Autodesk Fusion 360 part; units mm, degrees
note: some values were not read from the file. Set by a fixed rule: which sketch regions a step uses.
(part 14 of 15)
  line L11464 (261.515, -47.6876) -> (261.464, -47.4097)
  line L11465 (-56.9781, -48.1712) -> (-56.8353, -48.2894)
  line L11466 (-56.8353, -48.2894) -> (-56.7181, -48.4331)
  line L11467 (-57.5292, -49.9086) -> (-57.7133, -49.8866)
  line L11468 (-57.6874, -48.0256) -> (-57.5027, -48.0088)
  line L11469 (-57.7133, -49.8866) -> (-57.8897, -49.8293)
  line L11470 (264.04, -45.2787) -> (264.303, -45.3806)
  line L11471 (263.765, -45.2149) -> (264.04, -45.2787)
  line L11472 (-58.4437, -49.1303) -> (-58.4593, -48.9455)
  line L11473 (-56.631, -48.5968) -> (-56.5774, -48.7743)
  line L11474 (-57.1658, -49.8445) -> (-57.3444, -49.8943)
  line L11475 (-56.5593, -48.9588) -> (-56.5597, -48.9853)
  line L11476 (-58.4593, -48.9455) -> (-58.4386, -48.7613)
  line L11477 (-58.0295, -48.1639) -> (-57.8652, -48.078)
  line L11478 (94.3983, -48.4103) -> (94.5428, -48.2941)
  line L11479 (95.9894, -49.2995) -> (95.9308, -49.4755)
  line L11480 (264.775, -45.69) -> (264.973, -45.8914)
  line L11481 (-57.8897, -49.8293) -> (-58.0515, -49.7389)
  line L11482 (-57.3183, -48.0282) -> (-57.1412, -48.083)
  line L11483 (94.2791, -48.5523) -> (94.3983, -48.4103)
  line L11484 (72.3389, -48.542) -> (72.1284, -48.7305)
  line L11485 (261.453, -47.1274) -> (261.482, -46.8464)
  line L11486 (261.973, -45.8442) -> (262.177, -45.6492)
  line L11487 (263.201, -45.206) -> (263.483, -45.1905)
  line L11488 (264.678, -48.7706) -> (264.443, -48.9275)
  line L11489 (72.1284, -48.7305) -> (71.8935, -48.8875)
  line L11490 (265.432, -46.9085) -> (265.452, -47.1903)
  line L11491 (71.3695, -49.0949) -> (71.0908, -49.1413)
  line L11492 (69.9946, -48.9322) -> (69.7526, -48.7865)
  line L11493 (69.7526, -48.7865) -> (69.5335, -48.6081)
  line L11494 (72.9026, -47.1502) -> (72.8987, -47.2758)
  line L11495 (69.1811, -48.1683) -> (69.0548, -47.9156)
  line L11496 (69.1066, -46.2703) -> (69.2484, -46.026)
  line L11497 (262.924, -45.2612) -> (263.201, -45.206)
  line L11498 (265.141, -46.1186) -> (265.275, -46.3672)
  line L11499 (72.8232, -46.5922) -> (72.8827, -46.8684)
  line L11500 (262.177, -45.6492) -> (262.407, -45.485)
  line L11501 (265.275, -46.3672) -> (265.372, -46.6323)
  line L11502 (262.407, -45.485) -> (262.658, -45.3548)
  line L11503 (262.302, -48.8266) -> (262.083, -48.6482)
  line L11504 (70.1083, -45.3147) -> (70.3749, -45.2211)
  line L11505 (70.5278, -49.1148) -> (70.2548, -49.0424)
  line L11506 (70.6519, -45.166) -> (70.934, -45.1505)
  line L11507 (265.334, -47.8677) -> (265.219, -48.1261)
  line L11508 (71.7542, -45.3406) -> (72.0007, -45.4786)
  line L11509 (263.483, -45.1905) -> (263.765, -45.2149)
  line L11510 (72.8827, -46.8684) -> (72.9026, -47.1502)
  line L11511 (72.2252, -45.65) -> (72.4234, -45.8513)
  line L11512 (262.544, -48.9723) -> (262.302, -48.8266)
  line L11513 (70.8084, -49.148) -> (70.5278, -49.1148)
  line L11514 (68.9324, -46.8063) -> (69.0005, -46.5322)
  line L11515 (72.7254, -46.3272) -> (72.8232, -46.5922)
  line L11516 (258.64, -47.1418) -> (258.817, -47.1966)
  line L11517 (69.4233, -45.8042) -> (69.6278, -45.6092)
  line L11518 (68.9654, -47.6476) -> (68.9147, -47.3697)
  line L11519 (70.934, -45.1505) -> (71.2155, -45.1748)
  line L11520 (264.188, -49.0498) -> (263.919, -49.135)
  line L11521 (265.372, -46.6323) -> (265.432, -46.9085)
  line L11522 (72.4234, -45.8513) -> (72.5913, -46.0785)
  line L11523 (265.07, -48.3658) -> (264.888, -48.5821)
  line L11524 (71.8935, -48.8875) -> (71.6389, -49.0098)
  line L11525 (71.6389, -49.0098) -> (71.3695, -49.0949)
  line L11526 (261.656, -46.3104) -> (261.798, -46.0661)
  line L11527 (71.2155, -45.1748) -> (71.4907, -45.2386)
  line L11528 (72.7844, -47.8277) -> (72.6701, -48.0861)
  line L11529 (71.0908, -49.1413) -> (70.8084, -49.148)
  line L11530 (261.55, -46.5722) -> (261.656, -46.3104)
  line L11531 (72.6701, -48.0861) -> (72.5206, -48.3258)
  line L11532 (261.798, -46.0661) -> (261.973, -45.8442)
  line L11533 (69.3417, -48.4007) -> (69.1811, -48.1683)
  line L11534 (70.2548, -49.0424) -> (69.9946, -48.9322)
  line L11535 (258.98, -47.2848) -> (259.123, -47.403)
  line L11536 (72.0007, -45.4786) -> (72.2252, -45.65)
  line L11537 (265.452, -47.1903) -> (265.448, -47.3159)
  line L11538 (68.9036, -47.0874) -> (68.9324, -46.8063)
  line L11539 (261.482, -46.8464) -> (261.55, -46.5722)
  line L11540 (262.658, -45.3548) -> (262.924, -45.2612)
  line L11541 (68.9147, -47.3697) -> (68.9036, -47.0874)
  line L11542 (264.888, -48.5821) -> (264.678, -48.7706)
  line L11543 (72.8987, -47.2758) -> (72.8611, -47.5558)
  line L11544 (71.4907, -45.2386) -> (71.7542, -45.3406)
  line L11545 (72.5206, -48.3258) -> (72.3389, -48.542)
  line L11546 (72.5913, -46.0785) -> (72.7254, -46.3272)
  line L11547 (72.8611, -47.5558) -> (72.7844, -47.8277)
  line L11548 (76.4367, -47.2448) -> (76.5795, -47.3629)
  line L11549 (258.245, -49.0002) -> (258.069, -48.9429)
  line L11550 (257.784, -47.3937) -> (257.929, -47.2775)
  line L11551 (257.907, -48.8525) -> (257.766, -48.7323)
  line L11552 (258.614, -49.008) -> (258.429, -49.0222)
  line L11553 (258.817, -47.1966) -> (258.98, -47.2848)
  line L11554 (70.3749, -45.2211) -> (70.6519, -45.166)
  line L11555 (76.0965, -47.1017) -> (76.2736, -47.1566)
  line L11556 (69.2484, -46.026) -> (69.4233, -45.8042)
  line L11557 (76.2736, -47.1566) -> (76.4367, -47.2448)
  line L11558 (75.7274, -47.0992) -> (75.9121, -47.0824)
  line L11559 (75.2407, -47.3536) -> (75.3852, -47.2374)
  line L11560 (75.9121, -47.0824) -> (76.0965, -47.1017)
  line L11561 (283.011, -44.6584) -> (283.286, -44.7222)
  line L11562 (257.929, -47.2775) -> (258.093, -47.1916)
  line L11563 (74.9762, -47.8348) -> (75.0323, -47.6581)
  line L11564 (76.8373, -47.8478) -> (76.8554, -48.0323)
  line L11565 (257.576, -47.6982) -> (257.665, -47.5357)
  line L11566 (257.515, -48.2439) -> (257.499, -48.0591)
  line L11567 (258.429, -49.0222) -> (258.245, -49.0002)
  line L11568 (76.249, -48.918) -> (76.0704, -48.9679)
  line L11569 (259.381, -47.8879) -> (259.399, -48.0724)
  line L11570 (75.1069, -48.547) -> (75.0221, -48.3821)
  line L11571 (75.5496, -47.1515) -> (75.7274, -47.0992)
  line L11572 (74.9555, -48.0191) -> (74.9762, -47.8348)
  line L11573 (257.665, -47.5357) -> (257.784, -47.3937)
  line L11574 (283.286, -44.7222) -> (283.549, -44.8242)
  line L11575 (283.549, -44.8242) -> (283.796, -44.9622)
  line L11576 (76.8318, -48.2428) -> (76.7733, -48.4187)
  line L11577 (76.8551, -48.0589) -> (76.8318, -48.2428)
  line L11578 (69.6278, -45.6092) -> (69.8576, -45.4449)
  line L11579 (257.566, -48.4221) -> (257.515, -48.2439)
  line L11580 (257.651, -48.587) -> (257.566, -48.4221)
  line L11581 (259.375, -48.2829) -> (259.317, -48.4588)
  line L11582 (76.5795, -47.3629) -> (76.6967, -47.5066)
  line L11583 (258.958, -48.8745) -> (258.793, -48.9581)
  line L11584 (257.52, -47.8749) -> (257.576, -47.6982)
  line L11585 (69.5335, -48.6081) -> (69.3417, -48.4007)
  line L11586 (69.0548, -47.9156) -> (68.9654, -47.6476)
  line L11587 (258.093, -47.1916) -> (258.271, -47.1392)
  line L11588 (259.104, -48.7604) -> (258.958, -48.8745)
  line L11589 (258.069, -48.9429) -> (257.907, -48.8525)
  line L11590 (259.225, -48.62) -> (259.104, -48.7604)
  line L11591 (257.499, -48.0591) -> (257.52, -47.8749)
  line L11592 (76.0704, -48.9679) -> (75.8855, -48.9821)
  line L11593 (259.24, -47.5467) -> (259.327, -47.7104)
  line L11594 (69.8576, -45.4449) -> (70.1083, -45.3147)
  line L11595 (259.317, -48.4588) -> (259.225, -48.62)
  line L11596 (257.766, -48.7323) -> (257.651, -48.587)
  line L11597 (76.8554, -48.0323) -> (76.8551, -48.0589)
  line L11598 (258.456, -47.1224) -> (258.64, -47.1418)
  line L11599 (74.971, -48.2038) -> (74.9555, -48.0191)
  line L11600 (75.0323, -47.6581) -> (75.1216, -47.4956)
  line L11601 (69.0005, -46.5322) -> (69.1066, -46.2703)
  line L11602 (75.0221, -48.3821) -> (74.971, -48.2038)
  line L11603 (75.1216, -47.4956) -> (75.2407, -47.3536)
  line L11604 (75.3852, -47.2374) -> (75.5496, -47.1515)
  line L11605 (75.7014, -48.9602) -> (75.5251, -48.9029)
  line L11606 (258.793, -48.9581) -> (258.614, -49.008)
  line L11607 (258.271, -47.1392) -> (258.456, -47.1224)
  line L11608 (259.327, -47.7104) -> (259.381, -47.8879)
  line L11609 (259.123, -47.403) -> (259.24, -47.5467)
  line L11610 (259.399, -48.0724) -> (259.399, -48.0989)
  line L11611 (259.399, -48.0989) -> (259.375, -48.2829)
  line L11612 (53.3455, -45.5221) -> (53.4797, -45.7707)
  line L11613 (53.1777, -45.2949) -> (53.3455, -45.5221)
  line L11614 (281.903, -44.7983) -> (282.17, -44.7047)
  line L11615 (75.3633, -48.8124) -> (75.2221, -48.6923)
  line L11616 (283.923, -48.2141) -> (283.689, -48.3711)
  line L11617 (284.134, -48.0257) -> (283.923, -48.2141)
  line L11618 (53.0931, -47.9856) -> (52.8827, -48.1741)
  line L11619 (75.8855, -48.9821) -> (75.7014, -48.9602)
  line L11620 (281.653, -44.9285) -> (281.903, -44.7983)
  line L11621 (284.678, -46.352) -> (284.698, -46.6338)
  line L11622 (281.218, -45.2878) -> (281.423, -45.0928)
  line L11623 (52.3931, -48.4533) -> (52.1237, -48.5385)
  line L11624 (52.1237, -48.5385) -> (51.8451, -48.5849)
  line L11625 (280.85, -47.3992) -> (280.76, -47.1312)
  line L11626 (76.7733, -48.4187) -> (76.6817, -48.5799)
  line L11627 (283.689, -48.3711) -> (283.434, -48.4934)
  line L11628 (281.423, -45.0928) -> (281.653, -44.9285)
  line L11629 (280.727, -46.29) -> (280.796, -46.0158)
  line L11630 (282.05, -48.526) -> (281.79, -48.4158)
  line L11631 (284.698, -46.6338) -> (284.694, -46.7594)
  line L11632 (76.6817, -48.5799) -> (76.5606, -48.7203)
  line L11633 (53.4797, -45.7707) -> (53.5774, -46.0358)
  line L11634 (284.02, -45.1336) -> (284.218, -45.3349)
  line L11635 (52.2449, -44.6822) -> (52.5084, -44.7841)
  line L11636 (281.329, -48.0918) -> (281.137, -47.8843)
  line L11637 (76.7837, -47.6703) -> (76.8373, -47.8478)
  line L11638 (282.886, -48.6249) -> (282.603, -48.6316)
  line L11639 (284.218, -45.3349) -> (284.386, -45.5622)
  line L11640 (280.976, -47.6519) -> (280.85, -47.3992)
  line L11641 (53.6369, -46.312) -> (53.6568, -46.5938)
  line L11642 (280.796, -46.0158) -> (280.902, -45.7539)
  line L11643 (283.165, -48.5786) -> (282.886, -48.6249)
  line L11644 (281.548, -48.2701) -> (281.329, -48.0918)
  line L11645 (53.5774, -46.0358) -> (53.6369, -46.312)
  line L11646 (281.79, -48.4158) -> (281.548, -48.2701)
  line L11647 (284.465, -47.5697) -> (284.316, -47.8094)
  line L11648 (284.52, -45.8108) -> (284.618, -46.0758)
  line L11649 (280.71, -46.8533) -> (280.699, -46.571)
  line L11650 (52.6478, -48.331) -> (52.3931, -48.4533)
  line L11651 (284.316, -47.8094) -> (284.134, -48.0257)
  line L11652 (284.579, -47.3113) -> (284.465, -47.5697)
  line L11653 (284.618, -46.0758) -> (284.678, -46.352)
  line L11654 (283.434, -48.4934) -> (283.165, -48.5786)
  line L11655 (281.137, -47.8843) -> (280.976, -47.6519)
  line L11656 (283.796, -44.9622) -> (284.02, -45.1336)
  line L11657 (52.8827, -48.1741) -> (52.6478, -48.331)
  line L11658 (284.386, -45.5622) -> (284.52, -45.8108)
  line L11659 (280.699, -46.571) -> (280.727, -46.29)
  line L11660 (280.902, -45.7539) -> (281.043, -45.5097)
  line L11661 (76.6967, -47.5066) -> (76.7837, -47.6703)
  line L11662 (75.5251, -48.9029) -> (75.3633, -48.8124)
  line L11663 (282.17, -44.7047) -> (282.447, -44.6496)
  line L11664 (284.694, -46.7594) -> (284.656, -47.0394)
  line L11665 (53.4244, -47.5296) -> (53.2749, -47.7693)
  line L11666 (75.2221, -48.6923) -> (75.1069, -48.547)
  line L11667 (51.8451, -48.5849) -> (51.5626, -48.5915)
  line L11668 (53.2749, -47.7693) -> (53.0931, -47.9856)
  line L11669 (76.4145, -48.8344) -> (76.249, -48.918)
  line L11670 (53.5386, -47.2712) -> (53.4244, -47.5296)
  line L11671 (282.323, -48.5984) -> (282.05, -48.526)
  line L11672 (280.76, -47.1312) -> (280.71, -46.8533)
  line L11673 (76.5606, -48.7203) -> (76.4145, -48.8344)
  line L11674 (284.656, -47.0394) -> (284.579, -47.3113)
  line L11675 (282.603, -48.6316) -> (282.323, -48.5984)
  line L11676 (282.729, -44.6341) -> (283.011, -44.6584)
  line L11677 (52.9795, -45.0935) -> (53.1777, -45.2949)
  line L11678 (278.063, -46.6402) -> (278.226, -46.7284)
  line L11679 (49.7197, -47.0911) -> (49.6689, -46.8132)
  line L11680 (278.627, -47.3314) -> (278.645, -47.516)
  line L11681 (52.5084, -44.7841) -> (52.7549, -44.9221)
  line L11682 (278.369, -46.8466) -> (278.486, -46.9902)
  line L11683 (49.6578, -46.5309) -> (49.6866, -46.2499)
  line L11684 (51.1291, -44.6646) -> (51.4062, -44.6095)
  line L11685 (51.2821, -48.5583) -> (51.009, -48.4859)
  line L11686 (278.573, -47.1539) -> (278.627, -47.3314)
  line L11687 (278.645, -47.516) -> (278.644, -47.5425)
  line L11688 (50.6118, -44.8885) -> (50.8625, -44.7582)
  line L11689 (53.6568, -46.5938) -> (53.6529, -46.7193)
  line L11690 (50.8625, -44.7582) -> (51.1291, -44.6646)
  line L11691 (277.491, -48.4438) -> (277.315, -48.3865)
  line L11692 (278.471, -48.0636) -> (278.35, -48.2039)
  line L11693 (50.0027, -45.4696) -> (50.1776, -45.2477)
  line L11694 (276.822, -47.1417) -> (276.911, -46.9792)
  line L11695 (277.86, -48.4515) -> (277.675, -48.4657)
  line L11696 (57.3338, -46.8065) -> (57.4509, -46.9502)
  line L11697 (281.043, -45.5097) -> (281.218, -45.2878)
  line L11698 (276.745, -47.5027) -> (276.766, -47.3184)
  line L11699 (57.4509, -46.9502) -> (57.538, -47.1139)
  line L11700 (277.675, -48.4657) -> (277.491, -48.4438)
  line L11701 (49.6866, -46.2499) -> (49.7547, -45.9757)
  line L11702 (277.175, -46.721) -> (277.339, -46.6351)
  line L11703 (276.896, -48.0306) -> (276.812, -47.8657)
  line L11704 (52.7549, -44.9221) -> (52.9795, -45.0935)
  line L11705 (57.538, -47.1139) -> (57.5916, -47.2914)
  line L11706 (50.7489, -48.3758) -> (50.5068, -48.2301)
  line L11707 (49.8608, -45.7139) -> (50.0027, -45.4696)
  line L11708 (276.76, -47.6875) -> (276.745, -47.5027)
  line L11709 (51.6883, -44.594) -> (51.9697, -44.6184)
  line L11710 (278.644, -47.5425) -> (278.621, -47.7264)
  line L11711 (278.621, -47.7264) -> (278.563, -47.9024)
  line L11712 (49.7547, -45.9757) -> (49.8608, -45.7139)
  line L11713 (50.1776, -45.2477) -> (50.382, -45.0527)
  line L11714 (53.6153, -46.9993) -> (53.5386, -47.2712)
  line L11715 (50.096, -47.8442) -> (49.9354, -47.6118)
  line L11716 (49.6689, -46.8132) -> (49.6578, -46.5309)
  line L11717 (278.486, -46.9902) -> (278.573, -47.1539)
  line L11718 (50.2878, -48.0517) -> (50.096, -47.8442)
  line L11719 (278.038, -48.4017) -> (277.86, -48.4515)
  line L11720 (277.517, -46.5828) -> (277.701, -46.566)
  line L11721 (53.6529, -46.7193) -> (53.6153, -46.9993)
  line L11722 (50.5068, -48.2301) -> (50.2878, -48.0517)
  line L11723 (51.5626, -48.5915) -> (51.2821, -48.5583)
  line L11724 (51.009, -48.4859) -> (50.7489, -48.3758)
  line L11725 (277.339, -46.6351) -> (277.517, -46.5828)
  line L11726 (276.911, -46.9792) -> (277.03, -46.8372)
  line L11727 (57.5916, -47.2914) -> (57.6097, -47.4759)
  line L11728 (57.6097, -47.4759) -> (57.6093, -47.5024)
  line L11729 (49.8091, -47.3591) -> (49.7197, -47.0911)
  line L11730 (276.766, -47.3184) -> (276.822, -47.1417)
  line L11731 (278.35, -48.2039) -> (278.204, -48.3181)
  line L11732 (282.447, -44.6496) -> (282.729, -44.6341)
  line L11733 (57.1909, -46.6883) -> (57.3338, -46.8065)
  line L11734 (49.9354, -47.6118) -> (49.8091, -47.3591)
  line L11735 (278.226, -46.7284) -> (278.369, -46.8466)
  line L11736 (51.9697, -44.6184) -> (52.2449, -44.6822)
  line L11737 (51.4062, -44.6095) -> (51.6883, -44.594)
  line L11738 (277.886, -46.5854) -> (278.063, -46.6402)
  line L11739 (50.382, -45.0527) -> (50.6118, -44.8885)
  line L11740 (56.6663, -46.5259) -> (56.8507, -46.5453)
  line L11741 (57.3148, -48.1639) -> (57.1687, -48.278)
  line L11742 (55.7253, -47.6474) -> (55.7098, -47.4626)
  line L11743 (56.6398, -48.4257) -> (56.4557, -48.4037)
  line L11744 (55.7865, -47.1016) -> (55.8758, -46.9392)
  line L11745 (56.1395, -46.681) -> (56.3038, -46.5951)
  line L11746 (248.363, -47.5364) -> (248.347, -47.3516)
  line L11747 (55.9763, -48.1358) -> (55.8611, -47.9905)
  line L11748 (249.952, -48.0528) -> (249.806, -48.167)
  line L11749 (249.462, -48.3004) -> (249.277, -48.3147)
  line L11750 (249.488, -46.4343) -> (249.665, -46.4891)
  line L11751 (248.424, -46.9906) -> (248.513, -46.8281)
  line L11752 (249.641, -48.2506) -> (249.462, -48.3004)
  line L11753 (248.917, -48.2354) -> (248.755, -48.145)
  line L11754 (249.119, -46.4317) -> (249.304, -46.4149)
  line L11755 (248.499, -47.8795) -> (248.414, -47.7146)
  line L11756 (249.093, -48.2927) -> (248.917, -48.2354)
  line L11757 (248.368, -47.1673) -> (248.424, -46.9906)
  line L11758 (250.088, -46.8391) -> (250.175, -47.0028)
  line L11759 (249.806, -48.167) -> (249.641, -48.2506)
  line L11760 (248.513, -46.8281) -> (248.632, -46.6861)
  line L11761 (250.247, -47.3914) -> (250.224, -47.5753)
  line L11762 (85.2484, -46.3942) -> (85.4255, -46.449)
  line L11763 (277.315, -48.3865) -> (277.153, -48.2961)
  line L11764 (249.828, -46.5773) -> (249.971, -46.6955)
  line L11765 (56.8507, -46.5453) -> (57.0278, -46.6001)
  line L11766 (249.971, -46.6955) -> (250.088, -46.8391)
  line L11767 (248.755, -48.145) -> (248.614, -48.0248)
  line L11768 (248.632, -46.6861) -> (248.777, -46.5699)
  line L11769 (56.1175, -48.256) -> (55.9763, -48.1358)
  line L11770 (55.7764, -47.8256) -> (55.7253, -47.6474)
  line L11771 (250.073, -47.9125) -> (249.952, -48.0528)
  line L11772 (249.665, -46.4891) -> (249.828, -46.5773)
  line L11773 (248.777, -46.5699) -> (248.941, -46.484)
  line L11774 (57.0032, -48.3616) -> (56.8246, -48.4115)
  line L11775 (248.414, -47.7146) -> (248.363, -47.5364)
  line L11776 (57.5275, -47.8623) -> (57.436, -48.0235)
  line L11777 (277.03, -46.8372) -> (277.175, -46.721)
  line L11778 (277.153, -48.2961) -> (277.011, -48.1759)
  line L11779 (57.5861, -47.6864) -> (57.5275, -47.8623)
  line L11780 (57.1687, -48.278) -> (57.0032, -48.3616)
  line L11781 (277.011, -48.1759) -> (276.896, -48.0306)
  line L11782 (56.2793, -48.3464) -> (56.1175, -48.256)
  line L11783 (56.8246, -48.4115) -> (56.6398, -48.4257)
  line L11784 (55.7098, -47.4626) -> (55.7304, -47.2784)
  line L11785 (56.4557, -48.4037) -> (56.2793, -48.3464)
  line L11786 (57.436, -48.0235) -> (57.3148, -48.1639)
  line L11787 (278.204, -48.3181) -> (278.038, -48.4017)
  line L11788 (278.563, -47.9024) -> (278.471, -48.0636)
  line L11789 (57.0278, -46.6001) -> (57.1909, -46.6883)
  line L11790 (276.812, -47.8657) -> (276.76, -47.6875)
  line L11791 (56.4817, -46.5427) -> (56.6663, -46.5259)
  line L11792 (55.8611, -47.9905) -> (55.7764, -47.8256)
  line L11793 (55.995, -46.7971) -> (56.1395, -46.681)
  line L11794 (250.175, -47.0028) -> (250.229, -47.1803)
  line L11795 (55.7304, -47.2784) -> (55.7865, -47.1016)
  line L11796 (250.229, -47.1803) -> (250.247, -47.3649)
  line L11797 (248.941, -46.484) -> (249.119, -46.4317)
  line L11798 (250.247, -47.3649) -> (250.247, -47.3914)
  line L11799 (57.6093, -47.5024) -> (57.5861, -47.6864)
  line L11800 (248.614, -48.0248) -> (248.499, -47.8795)
  line L11801 (56.3038, -46.5951) -> (56.4817, -46.5427)
  line L11802 (277.701, -46.566) -> (277.886, -46.5854)
  line L11803 (55.8758, -46.9392) -> (55.995, -46.7971)
  line L11804 (269.404, -46.3347) -> (269.381, -46.5186)
  line L11805 (84.1842, -46.9506) -> (84.2735, -46.7881)
  line L11806 (267.771, -46.9681) -> (267.656, -46.8228)
  line L11807 (249.304, -46.4149) -> (249.488, -46.4343)
  line L11808 (85.4009, -48.2105) -> (85.2223, -48.2604)
  line L11809 (84.7015, -46.444) -> (84.8793, -46.3916)
  line L11810 (268.461, -45.3582) -> (268.646, -45.3775)
  line L11811 (85.4255, -46.449) -> (85.5886, -46.5372)
  line L11812 (66.0908, -45.3375) -> (66.2679, -45.3923)
  line L11813 (85.7314, -46.6554) -> (85.8486, -46.7991)
  line L11814 (268.435, -47.2579) -> (268.251, -47.236)
  line L11815 (66.2679, -45.3923) -> (66.431, -45.4805)
  line L11816 (66.431, -45.4805) -> (66.5739, -45.5987)
  line L11817 (86.0073, -47.3248) -> (86.007, -47.3513)
  line L11818 (84.5152, -48.1049) -> (84.374, -47.9847)
  line L11819 (66.5739, -45.5987) -> (66.6911, -45.7423)
  line L11820 (84.174, -47.6745) -> (84.1229, -47.4963)
  line L11821 (84.1281, -47.1273) -> (84.1842, -46.9506)
  line L11822 (85.9252, -47.7112) -> (85.8336, -47.8724)
  line L11823 (85.7125, -48.0128) -> (85.5664, -48.1269)
  line L11824 (250.165, -47.7513) -> (250.073, -47.9125)
  line L11825 (267.656, -46.8228) -> (267.571, -46.6579)
  line L11826 (85.2223, -48.2604) -> (85.0374, -48.2746)
  line L11827 (267.79, -45.6294) -> (267.935, -45.5132)
  line L11828 (84.2735, -46.7881) -> (84.3927, -46.646)
  line L11829 (85.9892, -47.1403) -> (86.0073, -47.3248)
  line L11830 (84.677, -48.1953) -> (84.5152, -48.1049)
  line L11831 (85.8336, -47.8724) -> (85.7125, -48.0128)
  line L11832 (84.374, -47.9847) -> (84.2588, -47.8394)
  line L11833 (269.246, -45.7824) -> (269.333, -45.9461)
  line L11834 (85.064, -46.3748) -> (85.2484, -46.3942)
  line L11835 (84.8533, -48.2526) -> (84.677, -48.1953)
  line L11836 (85.5664, -48.1269) -> (85.4009, -48.2105)
  line L11837 (269.333, -45.9461) -> (269.387, -46.1236)
  line L11838 (85.0374, -48.2746) -> (84.8533, -48.2526)
  line L11839 (85.8486, -46.7991) -> (85.9356, -46.9628)
  line L11840 (248.347, -47.3516) -> (248.368, -47.1673)
  line L11841 (268.823, -45.4324) -> (268.986, -45.5206)
  line L11842 (267.571, -46.6579) -> (267.52, -46.4796)
  line L11843 (269.129, -45.6387) -> (269.246, -45.7824)
  line L11844 (249.277, -48.3147) -> (249.093, -48.2927)
  line L11845 (84.1074, -47.3115) -> (84.1281, -47.1273)
  line L11846 (86.007, -47.3513) -> (85.9837, -47.5353)
  line L11847 (84.1229, -47.4963) -> (84.1074, -47.3115)
  line L11848 (84.8793, -46.3916) -> (85.064, -46.3748)
  line L11849 (269.387, -46.1236) -> (269.405, -46.3081)
  line L11850 (85.9356, -46.9628) -> (85.9892, -47.1403)
  line L11851 (84.5371, -46.5299) -> (84.7015, -46.444)
  line L11852 (269.11, -46.9961) -> (268.964, -47.1102)
  line L11853 (85.5886, -46.5372) -> (85.7314, -46.6554)
  line L11854 (269.381, -46.5186) -> (269.323, -46.6945)
  line L11855 (267.52, -46.4796) -> (267.505, -46.2949)
  line L11856 (268.646, -45.3775) -> (268.823, -45.4324)
  line L11857 (269.231, -46.8557) -> (269.11, -46.9961)
  line L11858 (267.935, -45.5132) -> (268.099, -45.4273)
  line L11859 (267.505, -46.2949) -> (267.525, -46.1106)
  line L11860 (268.099, -45.4273) -> (268.277, -45.375)
  line L11861 (268.277, -45.375) -> (268.461, -45.3582)
  line L11862 (269.323, -46.6945) -> (269.231, -46.8557)
  line L11863 (84.2588, -47.8394) -> (84.174, -47.6745)
  line L11864 (84.3927, -46.646) -> (84.5371, -46.5299)
  line L11865 (250.224, -47.5753) -> (250.165, -47.7513)
  line L11866 (85.9837, -47.5353) -> (85.9252, -47.7112)
  line L11867 (268.986, -45.5206) -> (269.129, -45.6387)
  line L11868 (65.5439, -45.3872) -> (65.7218, -45.3349)
  line L11869 (287.681, -46.7015) -> (287.496, -46.6795)
  line L11870 (288.632, -45.5672) -> (288.65, -45.7517)
  line L11871 (65.2164, -46.928) -> (65.1012, -46.7827)
  line L11872 (66.8498, -46.2681) -> (66.8494, -46.2946)
  line L11873 (66.2433, -47.1538) -> (66.0648, -47.2036)
  line L11874 (288.65, -45.7517) -> (288.65, -45.7782)
  line L11875 (66.8317, -46.0835) -> (66.8498, -46.2681)
  line L11876 (287.017, -46.4116) -> (286.902, -46.2663)
  line L11877 (66.5549, -46.956) -> (66.4088, -47.0702)
  line L11878 (288.568, -46.1381) -> (288.477, -46.2993)
  line L11879 (288.356, -46.4397) -> (288.21, -46.5538)
  line L11880 (286.917, -45.215) -> (287.036, -45.0729)
  line L11881 (65.2351, -45.5893) -> (65.3796, -45.4731)
  line L11882 (269.405, -46.3081) -> (269.404, -46.3347)
  line L11883 (66.0648, -47.2036) -> (65.8799, -47.2179)
  line L11884 (288.579, -45.3897) -> (288.632, -45.5672)
  line L11885 (267.671, -45.7714) -> (267.79, -45.6294)
  line L11886 (65.6958, -47.1959) -> (65.5195, -47.1386)
  line L11887 (65.1159, -45.7314) -> (65.2351, -45.5893)
  line L11888 (65.0165, -46.6178) -> (64.9654, -46.4396)
  line L11889 (288.492, -45.226) -> (288.579, -45.3897)
  line L11890 (288.232, -44.9641) -> (288.375, -45.0823)
  line L11891 (288.65, -45.7782) -> (288.627, -45.9622)
  line L11892 (65.3796, -45.4731) -> (65.5439, -45.3872)
  line L11893 (268.251, -47.236) -> (268.074, -47.1787)
  line L11894 (66.8262, -46.4785) -> (66.7677, -46.6545)
  line L11895 (288.069, -44.8759) -> (288.232, -44.9641)
  line L11896 (267.913, -47.0882) -> (267.771, -46.9681)
  line L11897 (287.865, -46.6873) -> (287.681, -46.7015)
  line L11898 (288.21, -46.5538) -> (288.044, -46.6374)
  line L11899 (66.4088, -47.0702) -> (66.2433, -47.1538)
  line L11900 (66.7781, -45.9061) -> (66.8317, -46.0835)
  line L11901 (287.158, -46.5318) -> (287.017, -46.4116)
  line L11902 (287.892, -44.8211) -> (288.069, -44.8759)
  line L11903 (64.9654, -46.4396) -> (64.9499, -46.2548)
  line L11904 (65.0266, -45.8938) -> (65.1159, -45.7314)
  line L11905 (65.7218, -45.3349) -> (65.9064, -45.3181)
  line L11906 (286.817, -46.1014) -> (286.766, -45.9232)
  line L11907 (65.5195, -47.1386) -> (65.3576, -47.0482)
  line L11908 (66.6761, -46.8157) -> (66.5549, -46.956)
  line L11909 (65.9064, -45.3181) -> (66.0908, -45.3375)
  line L11910 (47.0222, -44.8359) -> (47.1853, -44.924)
  line L11911 (65.8799, -47.2179) -> (65.6958, -47.1959)
  line L11912 (64.9499, -46.2548) -> (64.9705, -46.0706)
  line L11913 (288.044, -46.6374) -> (287.865, -46.6873)
  line L11914 (64.9705, -46.0706) -> (65.0266, -45.8938)
  line L11915 (66.6911, -45.7423) -> (66.7781, -45.9061)
  line L11916 (286.902, -46.2663) -> (286.817, -46.1014)
  line L11917 (267.525, -46.1106) -> (267.582, -45.9339)
  line L11918 (65.3576, -47.0482) -> (65.2164, -46.928)
  line L11919 (288.477, -46.2993) -> (288.356, -46.4397)
  line L11920 (268.62, -47.2437) -> (268.435, -47.2579)
  line L11921 (65.1012, -46.7827) -> (65.0165, -46.6178)
  line L11922 (268.074, -47.1787) -> (267.913, -47.0882)
  line L11923 (286.771, -45.5542) -> (286.827, -45.3774)
  line L11924 (287.32, -46.6222) -> (287.158, -46.5318)
  line L11925 (268.798, -47.1938) -> (268.62, -47.2437)
  line L11926 (287.036, -45.0729) -> (287.18, -44.9568)
  line L11927 (287.345, -44.8709) -> (287.522, -44.8185)
  line L11928 (66.7677, -46.6545) -> (66.6761, -46.8157)
  line L11929 (267.582, -45.9339) -> (267.671, -45.7714)
  line L11930 (66.8494, -46.2946) -> (66.8262, -46.4785)
  line L11931 (268.964, -47.1102) -> (268.798, -47.1938)
  line L11932 (-41.4665, -46.0435) -> (-41.7312, -46.0876)
  line L11933 (287.522, -44.8185) -> (287.707, -44.8017)
  line L11934 (47.6037, -45.7382) -> (47.5804, -45.9221)
  line L11935 (45.7248, -45.5141) -> (45.7808, -45.3374)
  line L11936 (46.45, -46.6395) -> (46.2737, -46.5822)
  line L11937 (-42.266, -46.0623) -> (-42.5254, -45.9936)
  line L11938 (47.3092, -46.3996) -> (47.1631, -46.5137)
  line L11939 (-41.3513, -42.38) -> (-41.101, -42.4768)
  line L11940 (-41.7312, -46.0876) -> (-41.9995, -46.0939)
  line L11941 (-40.4652, -42.962) -> (-40.3058, -43.1779)
  line L11942 (287.18, -44.9568) -> (287.345, -44.8709)
  line L11943 (45.8702, -45.1749) -> (45.9893, -45.0329)
  line L11944 (-42.7726, -45.8889) -> (-43.0025, -45.7505)
  line L11945 (-40.7455, -45.6973) -> (-40.9686, -45.8464)
  line L11946 (46.845, -44.781) -> (47.0222, -44.8359)
  line L11947 (-40.5456, -45.5182) -> (-40.7455, -45.6973)
  line L11948 (-40.0495, -44.5813) -> (-40.1223, -44.8396)
  line L11949 (47.5323, -45.3496) -> (47.5859, -45.5271)
  line L11950 (46.1118, -46.4917) -> (45.9706, -46.3716)
  line L11951 (45.7196, -45.8831) -> (45.7041, -45.6984)
  line L11952 (-40.1223, -44.8396) -> (-40.2308, -45.0851)
  line L11953 (-43.0025, -45.7505) -> (-43.2106, -45.581)
  line L11954 (-42.5254, -45.9936) -> (-42.7726, -45.8889)
  line L11955 (47.5804, -45.9221) -> (47.5219, -46.098)
  line L11956 (46.6607, -44.7616) -> (46.845, -44.781)
  line L11957 (-40.6535, -42.7708) -> (-40.4652, -42.962)
  line L11958 (46.476, -44.7785) -> (46.6607, -44.7616)
  line L11959 (-41.101, -42.4768) -> (-40.8669, -42.608)
  line L11960 (286.766, -45.9232) -> (286.751, -45.7384)
  line L11961 (47.1631, -46.5137) -> (46.9976, -46.5973)
  line L11962 (46.6341, -46.6614) -> (46.45, -46.6395)
  line L11963 (45.9706, -46.3716) -> (45.8555, -46.2262)
  line L11964 (45.9893, -45.0329) -> (46.1338, -44.9167)
  line L11965 (-40.01, -44.196) -> (-40.0137, -44.3153)
  line L11966 (46.9976, -46.5973) -> (46.819, -46.6472)
  line L11967 (-40.1783, -43.4141) -> (-40.0854, -43.6659)
  line L11968 (286.751, -45.7384) -> (286.771, -45.5542)
  line L11969 (46.2737, -46.5822) -> (46.1118, -46.4917)
  line L11970 (46.2981, -44.8308) -> (46.476, -44.7785)
  line L11971 (45.7707, -46.0613) -> (45.7196, -45.8831)
  line L11972 (46.819, -46.6472) -> (46.6341, -46.6614)
  line L11973 (-40.2308, -45.0851) -> (-40.3729, -45.3128)
  line L11974 (287.496, -46.6795) -> (287.32, -46.6222)
  line L11975 (47.1853, -44.924) -> (47.3281, -45.0422)
  line L11976 (-40.0137, -44.3153) -> (-40.0495, -44.5813)
  line L11977 (46.1338, -44.9167) -> (46.2981, -44.8308)
  line L11978 (288.375, -45.0823) -> (288.492, -45.226)
  line L11979 (-43.3928, -45.384) -> (-43.5454, -45.1632)
  line L11980 (47.5219, -46.098) -> (47.4303, -46.2592)
  line L11981 (-43.6654, -44.9231) -> (-43.7503, -44.6685)
  line L11982 (45.7808, -45.3374) -> (45.8702, -45.1749)
  line L11983 (-41.6128, -42.3194) -> (-41.3513, -42.38)
  line L11984 (45.8555, -46.2262) -> (45.7707, -46.0613)
  line L11985 (288.627, -45.9622) -> (288.568, -46.1381)
  line L11986 (286.827, -45.3774) -> (286.917, -45.215)
  line L11987 (287.707, -44.8017) -> (287.892, -44.8211)
  line L11988 (47.3281, -45.0422) -> (47.4453, -45.1859)
  line L11989 (47.5859, -45.5271) -> (47.604, -45.7116)
  line L11990 (45.7041, -45.6984) -> (45.7248, -45.5141)
  line L11991 (-40.0854, -43.6659) -> (-40.029, -43.9283)
  line L11992 (-40.3729, -45.3128) -> (-40.5456, -45.5182)
  line L11993 (47.4453, -45.1859) -> (47.5323, -45.3496)
  line L11994 (47.604, -45.7116) -> (47.6037, -45.7382)
  line L11995 (47.4303, -46.2592) -> (47.3092, -46.3996)
  line L11996 (-43.7817, -43.8693) -> (-43.717, -43.6089)
  line L11997 (300.413, -41.6205) -> (300.664, -41.4903)
  line L11998 (300.664, -41.4903) -> (300.931, -41.3967)
  line L11999 (-41.2106, -45.9626) -> (-41.4665, -46.0435)
  line L12000 (303.458, -43.3258) -> (303.454, -43.4514)
  line L12001 (300.183, -41.7848) -> (300.413, -41.6205)
  line L12002 (301.925, -45.2706) -> (301.646, -45.317)
  line L12003 (303.147, -42.2542) -> (303.281, -42.5028)
  line L12004 (299.488, -42.982) -> (299.556, -42.7078)
  line L12005 (-43.5454, -45.1632) -> (-43.6654, -44.9231)
  line L12006 (-43.717, -43.6089) -> (-43.6163, -43.3601)
  line L12007 (33.2091, -41.3104) -> (33.4843, -41.3742)
  line L12008 (33.9943, -41.6141) -> (34.2189, -41.7855)
  line L12009 (303.34, -44.0033) -> (303.226, -44.2617)
  line L12010 (303.438, -43.044) -> (303.458, -43.3258)
  line L12011 (299.897, -44.5763) -> (299.737, -44.3439)
  line L12012 (300.931, -41.3967) -> (301.208, -41.3416)
  line L12013 (302.684, -44.9061) -> (302.449, -45.0631)
  line L12014 (-42.4114, -42.3633) -> (-42.1481, -42.311)
  line L12015 (-43.7503, -44.6685) -> (-43.7985, -44.4045)
  line L12016 (-40.3058, -43.1779) -> (-40.1783, -43.4141)
  line L12017 (-43.8091, -44.1363) -> (-43.7817, -43.8693)
  line L12018 (302.046, -41.4142) -> (302.31, -41.5162)
  line L12019 (-42.6646, -42.4523) -> (-42.4114, -42.3633)
  line L12020 (-42.1481, -42.311) -> (-41.8802, -42.2962)
  line L12021 (302.194, -45.1854) -> (301.925, -45.2706)
  line L12022 (301.49, -41.3261) -> (301.771, -41.3504)
  line L12023 (301.083, -45.2904) -> (300.81, -45.218)
  line L12024 (-43.6163, -43.3601) -> (-43.4815, -43.128)
  line L12025 (299.737, -44.3439) -> (299.61, -44.0912)
  line L12026 (299.61, -44.0912) -> (299.521, -43.8232)
  line L12027 (-43.7985, -44.4045) -> (-43.8091, -44.1363)
  line L12028 (-43.1211, -42.732) -> (-42.9027, -42.576)
  line L12029 (299.979, -41.9798) -> (300.183, -41.7848)
  line L12030 (302.31, -41.5162) -> (302.556, -41.6542)
  line L12031 (-41.9995, -46.0939) -> (-42.266, -46.0623)
  line L12032 (-40.8669, -42.608) -> (-40.6535, -42.7708)
  line L12033 (302.979, -42.0269) -> (303.147, -42.2542)
  line L12034 (303.454, -43.4514) -> (303.417, -43.7314)
  line L12035 (301.646, -45.317) -> (301.364, -45.3236)
  line L12036 (-40.9686, -45.8464) -> (-41.2106, -45.9626)
  line L12037 (301.208, -41.3416) -> (301.49, -41.3261)
  line L12038 (300.089, -44.7838) -> (299.897, -44.5763)
  line L12039 (-42.9027, -42.576) -> (-42.6646, -42.4523)
  line L12040 (303.417, -43.7314) -> (303.34, -44.0033)
  line L12041 (300.81, -45.218) -> (300.55, -45.1078)
  line L12042 (-40.029, -43.9283) -> (-40.01, -44.196)
  line L12043 (301.771, -41.3504) -> (302.046, -41.4142)
  line L12044 (303.281, -42.5028) -> (303.379, -42.7678)
  line L12045 (-41.8802, -42.2962) -> (-41.6128, -42.3194)
  line L12046 (-43.3153, -42.9173) -> (-43.1211, -42.732)
  line L12047 (33.4843, -41.3742) -> (33.7478, -41.4761)
  line L12048 (303.076, -44.5014) -> (302.894, -44.7177)
  line L12049 (303.226, -44.2617) -> (303.076, -44.5014)
  line L12050 (302.556, -41.6542) -> (302.781, -41.8256)
  line L12051 (300.308, -44.9621) -> (300.089, -44.7838)
  line L12052 (302.894, -44.7177) -> (302.684, -44.9061)
  line L12053 (302.781, -41.8256) -> (302.979, -42.0269)
  line L12054 (301.364, -45.3236) -> (301.083, -45.2904)
  line L12055 (33.7478, -41.4761) -> (33.9943, -41.6141)
  line L12056 (303.379, -42.7678) -> (303.438, -43.044)
  line L12057 (-43.2106, -45.581) -> (-43.3928, -45.384)
  line L12058 (-43.4815, -43.128) -> (-43.3153, -42.9173)
  line L12059 (302.449, -45.0631) -> (302.194, -45.1854)
  line L12060 (30.926, -42.9419) -> (30.9941, -42.6677)
  line L12061 (34.4171, -41.9869) -> (34.5849, -42.2141)
  line L12062 (30.8972, -43.2229) -> (30.926, -42.9419)
  line L12063 (31.417, -41.9397) -> (31.6214, -41.7447)
  line L12064 (34.2189, -41.7855) -> (34.4171, -41.9869)
  line L12065 (34.7191, -42.4627) -> (34.8168, -42.7278)
  line L12066 (34.8168, -42.7278) -> (34.8763, -43.004)
  line L12067 (34.6638, -44.2216) -> (34.5143, -44.4613)
  line L12068 (31.7462, -44.9221) -> (31.5272, -44.7437)
  line L12069 (34.778, -43.9632) -> (34.6638, -44.2216)
  line L12070 (33.3631, -45.2305) -> (33.0845, -45.2769)
  line L12071 (297.405, -44.208) -> (297.405, -44.2345)
  line L12072 (31.8513, -41.5805) -> (32.102, -41.4503)
  line L12073 (31.5272, -44.7437) -> (31.3354, -44.5362)
  line L12074 (297.405, -44.2345) -> (297.382, -44.4184)
  line L12075 (31.6214, -41.7447) -> (31.8513, -41.5805)
  line L12076 (34.5849, -42.2141) -> (34.7191, -42.4627)
  line L12077 (299.521, -43.8232) -> (299.47, -43.5453)
  line L12078 (33.6325, -45.1453) -> (33.3631, -45.2305)
  line L12079 (32.3685, -41.3566) -> (32.6456, -41.3015)
  line L12080 (295.657, -44.7226) -> (295.572, -44.5577)
  line L12081 (33.0845, -45.2769) -> (32.802, -45.2835)
  line L12082 (30.9941, -42.6677) -> (31.1002, -42.4059)
  line L12083 (32.5215, -45.2503) -> (32.2484, -45.1779)
  line L12084 (299.556, -42.7078) -> (299.662, -42.4459)
  line L12085 (299.662, -42.4459) -> (299.804, -42.2017)
  line L12086 (295.521, -44.3795) -> (295.506, -44.1947)
  line L12087 (295.506, -44.1947) -> (295.526, -44.0104)
  line L12088 (30.9083, -43.5052) -> (30.8972, -43.2229)
  line L12089 (300.55, -45.1078) -> (300.308, -44.9621)
  line L12090 (31.3354, -44.5362) -> (31.1748, -44.3038)
  line L12091 (34.8923, -43.4113) -> (34.8547, -43.6913)
  line L12092 (32.9277, -41.286) -> (33.2091, -41.3104)
  line L12093 (295.772, -44.8679) -> (295.657, -44.7226)
  line L12094 (296.62, -45.1435) -> (296.436, -45.1578)
  line L12095 (296.436, -45.1578) -> (296.251, -45.1358)
  line L12096 (296.824, -43.3322) -> (296.987, -43.4204)
  line L12097 (31.9883, -45.0678) -> (31.7462, -44.9221)
  line L12098 (34.5143, -44.4613) -> (34.3325, -44.6776)
  line L12099 (299.459, -43.263) -> (299.488, -42.982)
  line L12100 (30.9591, -43.7831) -> (30.9083, -43.5052)
  line L12101 (296.251, -45.1358) -> (296.075, -45.0785)
  line L12102 (299.47, -43.5453) -> (299.459, -43.263)
  line L12103 (296.646, -43.2774) -> (296.824, -43.3322)
  line L12104 (34.3325, -44.6776) -> (34.1221, -44.8661)
  line L12105 (32.2484, -45.1779) -> (31.9883, -45.0678)
  line L12106 (34.8547, -43.6913) -> (34.778, -43.9632)
  line L12107 (33.8872, -45.023) -> (33.6325, -45.1453)
  line L12108 (34.1221, -44.8661) -> (33.8872, -45.023)
  line L12109 (296.075, -45.0785) -> (295.913, -44.9881)
  line L12110 (32.6456, -41.3015) -> (32.9277, -41.286)
  line L12111 (295.572, -44.5577) -> (295.521, -44.3795)
  line L12112 (296.987, -43.4204) -> (297.13, -43.5386)
  line L12113 (297.111, -44.8959) -> (296.964, -45.0101)
  line L12114 (296.799, -45.0937) -> (296.62, -45.1435)
  line L12115 (295.913, -44.9881) -> (295.772, -44.8679)
  line L12116 (31.1748, -44.3038) -> (31.0485, -44.0511)
  line L12117 (31.1002, -42.4059) -> (31.2421, -42.1616)
  line L12118 (31.2421, -42.1616) -> (31.417, -41.9397)
  line L12119 (299.804, -42.2017) -> (299.979, -41.9798)
  line L12120 (34.8963, -43.2858) -> (34.8923, -43.4113)
  line L12121 (32.802, -45.2835) -> (32.5215, -45.2503)
  line L12122 (31.0485, -44.0511) -> (30.9591, -43.7831)
  line L12123 (34.8763, -43.004) -> (34.8963, -43.2858)
  line L12124 (38.767, -44.5543) -> (38.6754, -44.7155)
  line L12125 (297.232, -44.7556) -> (297.111, -44.8959)
  line L12126 (38.831, -43.9834) -> (38.8491, -44.1679)
  line L12127 (296.277, -43.2748) -> (296.462, -43.258)
  line L12128 (307.252, -41.918) -> (307.339, -42.0817)
  line L12129 (307.237, -42.9913) -> (307.116, -43.1317)
  line L12130 (306.992, -41.6561) -> (307.135, -41.7743)
  line L12131 (307.329, -42.8301) -> (307.237, -42.9913)
  line L12132 (37.2344, -43.4891) -> (37.3789, -43.373)
  line L12133 (307.116, -43.1317) -> (306.97, -43.2458)
  line L12134 (297.387, -44.0234) -> (297.405, -44.208)
  line L12135 (307.387, -42.6542) -> (307.329, -42.8301)
  line L12136 (305.578, -42.7934) -> (305.527, -42.6152)
  line L12137 (307.135, -41.7743) -> (307.252, -41.918)
  line L12138 (306.829, -41.5679) -> (306.992, -41.6561)
  line L12139 (307.393, -42.2592) -> (307.411, -42.4437)
  line L12140 (306.805, -43.3294) -> (306.626, -43.3793)
  line L12141 (38.0901, -43.2373) -> (38.2672, -43.2921)
  line L12142 (295.791, -43.5292) -> (295.935, -43.413)
  line L12143 (38.5732, -43.4985) -> (38.6904, -43.6422)
  line L12144 (307.411, -42.4702) -> (307.387, -42.6542)
  line L12145 (306.652, -41.5131) -> (306.829, -41.5679)
  line L12146 (305.527, -42.6152) -> (305.511, -42.4304)
  line L12147 (295.526, -44.0104) -> (295.582, -43.8337)
  line L12148 (38.6904, -43.6422) -> (38.7774, -43.8059)
  line L12149 (37.1152, -43.6312) -> (37.2344, -43.4891)
  line L12150 (38.2426, -45.0536) -> (38.064, -45.1035)
  line L12151 (37.3789, -43.373) -> (37.5432, -43.2871)
  line L12152 (37.8792, -45.1177) -> (37.6951, -45.0957)
  line L12153 (38.5542, -44.8559) -> (38.4081, -44.97)
  line L12154 (37.3569, -44.948) -> (37.2157, -44.8278)
  line L12155 (295.672, -43.6712) -> (295.791, -43.5292)
  line L12156 (296.964, -45.0101) -> (296.799, -45.0937)
  line L12157 (37.1005, -44.6825) -> (37.0158, -44.5176)
  line L12158 (37.5187, -45.0384) -> (37.3569, -44.948)
  line L12159 (38.8487, -44.1944) -> (38.8255, -44.3784)
  line L12160 (297.382, -44.4184) -> (297.323, -44.5944)
  line L12161 (295.582, -43.8337) -> (295.672, -43.6712)
  line L12162 (296.1, -43.3271) -> (296.277, -43.2748)
  line L12163 (297.13, -43.5386) -> (297.247, -43.6822)
  line L12164 (38.4081, -44.97) -> (38.2426, -45.0536)
  line L12165 (36.9647, -44.3394) -> (36.9492, -44.1546)
  line L12166 (297.247, -43.6822) -> (297.334, -43.8459)
  line L12167 (306.97, -43.2458) -> (306.805, -43.3294)
  line L12168 (307.411, -42.4437) -> (307.411, -42.4702)
  line L12169 (295.935, -43.413) -> (296.1, -43.3271)
  line L12170 (306.257, -43.3715) -> (306.081, -43.3142)
  line L12171 (37.9057, -43.2179) -> (38.0901, -43.2373)
  line L12172 (38.8255, -44.3784) -> (38.767, -44.5543)
  line L12173 (307.339, -42.0817) -> (307.393, -42.2592)
  line L12174 (38.064, -45.1035) -> (37.8792, -45.1177)
  line L12175 (38.6754, -44.7155) -> (38.5542, -44.8559)
  line L12176 (37.2157, -44.8278) -> (37.1005, -44.6825)
  line L12177 (37.6951, -45.0957) -> (37.5187, -45.0384)
  line L12178 (38.4303, -43.3803) -> (38.5732, -43.4985)
  line L12179 (38.7774, -43.8059) -> (38.831, -43.9834)
  line L12180 (36.9492, -44.1546) -> (36.9698, -43.9704)
  line L12181 (296.462, -43.258) -> (296.646, -43.2774)
  line L12182 (38.2672, -43.2921) -> (38.4303, -43.3803)
  line L12183 (38.8491, -44.1679) -> (38.8487, -44.1944)
  line L12184 (37.0158, -44.5176) -> (36.9647, -44.3394)
  line L12185 (297.334, -43.8459) -> (297.387, -44.0234)
  line L12186 (32.102, -41.4503) -> (32.3685, -41.3566)
  line L12187 (297.323, -44.5944) -> (297.232, -44.7556)
  line L12188 (27.0949, -42.9183) -> (27.0101, -42.7533)
  line L12189 (305.778, -43.1036) -> (305.663, -42.9583)
  line L12190 (27.0101, -42.7533) -> (26.959, -42.5751)
  line L12191 (28.6697, -42.9512) -> (28.5486, -43.0916)
  line L12192 (37.7211, -43.2347) -> (37.9057, -43.2179)
  line L12193 (305.532, -42.2462) -> (305.588, -42.0694)
  line L12194 (28.5486, -43.0916) -> (28.4025, -43.2057)
  line L12195 (305.941, -41.6488) -> (306.105, -41.5629)
  line L12196 (306.468, -41.4937) -> (306.652, -41.5131)
  line L12197 (28.2616, -41.5279) -> (28.4247, -41.616)
  line L12198 (27.8735, -43.3534) -> (27.6894, -43.3315)
  line L12199 (7.3961, -39.0289) -> (7.6713, -39.0927)
  line L12200 (7.8195, -42.8639) -> (7.5501, -42.9491)
  line L12201 (28.8431, -42.4302) -> (28.8198, -42.6141)
  line L12202 (8.1813, -39.3327) -> (8.4059, -39.5041)
  line L12203 (7.5501, -42.9491) -> (7.2714, -42.9954)
  line L12204 (305.511, -42.4304) -> (305.532, -42.2462)
  line L12205 (37.0259, -43.7936) -> (37.1152, -43.6312)
  line L12206 (28.8434, -42.4036) -> (28.8431, -42.4302)
  line L12207 (26.9642, -42.2061) -> (27.0203, -42.0294)
  line L12208 (9.0417, -41.4099) -> (8.965, -41.6818)
  line L12209 (306.283, -41.5105) -> (306.468, -41.4937)
  line L12210 (28.4247, -41.616) -> (28.5675, -41.7342)
  line L12211 (8.906, -40.1813) -> (9.0038, -40.4463)
  line L12212 (306.626, -43.3793) -> (306.441, -43.3935)
  line L12213 (306.081, -43.3142) -> (305.919, -43.2238)
  line L12214 (36.9698, -43.9704) -> (37.0259, -43.7936)
  line L12215 (27.5376, -41.5228) -> (27.7154, -41.4705)
  line L12216 (27.2101, -43.0636) -> (27.0949, -42.9183)
  line L12217 (305.663, -42.9583) -> (305.578, -42.7934)
  line L12218 (28.5675, -41.7342) -> (28.6847, -41.8779)
  line L12219 (28.0584, -43.3392) -> (27.8735, -43.3534)
  line L12220 (27.2288, -41.7249) -> (27.3733, -41.6087)
  line L12221 (7.9348, -39.1947) -> (8.1813, -39.3327)
  line L12222 (26.959, -42.5751) -> (26.9435, -42.3904)
  line L12223 (7.2715, -42.9954) -> (6.989, -43.0021)
  line L12224 (26.9435, -42.3904) -> (26.9642, -42.2061)
  line L12225 (305.796, -41.7649) -> (305.941, -41.6488)
  line L12226 (305.588, -42.0694) -> (305.677, -41.907)
  line L12227 (37.5432, -43.2871) -> (37.7211, -43.2347)
  line L12228 (28.0845, -41.473) -> (28.2616, -41.5279)
  line L12229 (8.8508, -41.9402) -> (8.7013, -42.1799)
  line L12230 (305.919, -43.2238) -> (305.778, -43.1036)
  line L12231 (9.0633, -40.7225) -> (9.0832, -41.0043)
  line L12232 (27.6894, -43.3315) -> (27.5131, -43.2742)
  line L12233 (28.8198, -42.6141) -> (28.7613, -42.79)
  line L12234 (28.8253, -42.2191) -> (28.8434, -42.4036)
  line L12235 (28.7718, -42.0416) -> (28.8253, -42.2191)
  line L12236 (305.677, -41.907) -> (305.796, -41.7649)
  line L12237 (8.965, -41.6818) -> (8.8508, -41.9402)
  line L12238 (8.0741, -42.7416) -> (7.8195, -42.8639)
  line L12239 (8.309, -42.5846) -> (8.0741, -42.7416)
  line L12240 (27.7154, -41.4705) -> (27.9001, -41.4537)
  line L12241 (27.0203, -42.0294) -> (27.1096, -41.8669)
  line L12242 (9.0038, -40.4463) -> (9.0633, -40.7225)
  line L12243 (9.0793, -41.1299) -> (9.0417, -41.4099)
  line L12244 (27.5131, -43.2742) -> (27.3513, -43.1837)
  line L12245 (28.4025, -43.2057) -> (28.237, -43.2893)
  line L12246 (28.237, -43.2893) -> (28.0584, -43.3392)
  line L12247 (306.441, -43.3935) -> (306.257, -43.3715)
  line L12248 (306.105, -41.5629) -> (306.283, -41.5105)
  line L12249 (28.6847, -41.8779) -> (28.7718, -42.0416)
  line L12250 (27.3513, -43.1837) -> (27.2101, -43.0636)
  line L12251 (28.7613, -42.79) -> (28.6697, -42.9512)
  line L12252 (5.1461, -41.5017) -> (5.0953, -41.2238)
  line L12253 (2.6116, -39.3346) -> (2.7545, -39.4528)
  line L12254 (11.2875, -42.4011) -> (11.2028, -42.2362)
  line L12255 (11.1517, -42.0579) -> (11.1362, -41.8732)
  line L12256 (12.6173, -41.0989) -> (12.7601, -41.2171)
  line L12257 (5.3617, -42.0224) -> (5.2355, -41.7697)
  line L12258 (13.018, -41.7019) -> (13.0361, -41.8865)
  line L12259 (5.0842, -40.9415) -> (5.113, -40.6605)
  line L12260 (11.4027, -42.5464) -> (11.2875, -42.4011)
  line L12261 (2.9587, -39.7602) -> (3.0123, -39.9377)
  line L12262 (2.8717, -39.5965) -> (2.9587, -39.7602)
  line L12263 (13.0124, -42.0969) -> (12.9539, -42.2729)
  line L12264 (3.0304, -40.1222) -> (3.03, -40.1487)
  line L12265 (12.4542, -41.0107) -> (12.6173, -41.0989)
  line L12266 (5.5224, -42.2548) -> (5.3617, -42.0224)
  line L12267 (6.989, -43.0021) -> (6.7085, -42.9689)
  line L12268 (12.4296, -42.7722) -> (12.251, -42.822)
  line L12269 (8.4059, -39.5041) -> (8.6041, -39.7054)
  line L12270 (7.6713, -39.0927) -> (7.9348, -39.1947)
  line L12271 (8.6041, -39.7054) -> (8.7719, -39.9327)
  line L12272 (6.0382, -39.299) -> (6.2889, -39.1688)
  line L12273 (5.8084, -39.4633) -> (6.0382, -39.299)
  line L12274 (12.2771, -40.9559) -> (12.4542, -41.0107)
  line L12275 (11.2129, -41.5122) -> (11.3022, -41.3497)
  line L12276 (5.604, -39.6583) -> (5.8084, -39.4633)
  line L12277 (13.0361, -41.8865) -> (13.0357, -41.913)
  line L12278 (5.0953, -41.2238) -> (5.0842, -40.9415)
  line L12279 (5.4291, -39.8802) -> (5.604, -39.6583)
  line L12280 (12.0927, -40.9365) -> (12.2771, -40.9559)
  line L12281 (12.9539, -42.2729) -> (12.8623, -42.4341)
  line L12282 (8.7013, -42.1799) -> (8.5195, -42.3961)
  line L12283 (8.7719, -39.9327) -> (8.906, -40.1813)
  line L12284 (8.5195, -42.3961) -> (8.309, -42.5846)
  line L12285 (6.4354, -42.8965) -> (6.1753, -42.7863)
  line L12286 (12.8773, -41.3607) -> (12.9644, -41.5244)
  line L12287 (12.9644, -41.5244) -> (13.018, -41.7019)
  line L12288 (9.0832, -41.0043) -> (9.0793, -41.1299)
  line L12289 (5.1811, -40.3863) -> (5.2872, -40.1244)
  line L12290 (11.4214, -41.2077) -> (11.5659, -41.0915)
  line L12291 (6.1753, -42.7863) -> (5.9332, -42.6406)
  line L12292 (13.0357, -41.913) -> (13.0124, -42.0969)
  line L12293 (12.8623, -42.4341) -> (12.7412, -42.5744)
  line L12294 (27.1096, -41.8669) -> (27.2288, -41.7249)
  line L12295 (6.7085, -42.9689) -> (6.4354, -42.8965)
  line L12296 (6.2889, -39.1688) -> (6.5555, -39.0752)
  line L12297 (5.9332, -42.6406) -> (5.7141, -42.4623)
  line L12298 (5.2355, -41.7697) -> (5.1461, -41.5017)
  line L12299 (7.1147, -39.0046) -> (7.3961, -39.0289)
  line L12300 (5.7141, -42.4623) -> (5.5224, -42.2548)
  line L12301 (2.7545, -39.4528) -> (2.8717, -39.5965)
  line L12302 (11.1568, -41.6889) -> (11.2129, -41.5122)
  line L12303 (12.251, -42.822) -> (12.0662, -42.8362)
  line L12304 (5.2872, -40.1244) -> (5.4291, -39.8802)
  line L12305 (2.2714, -39.1916) -> (2.4486, -39.2464)
  line L12306 (5.113, -40.6605) -> (5.1811, -40.3863)
  line L12307 (11.1362, -41.8732) -> (11.1568, -41.6889)
  line L12308 (3.0123, -39.9377) -> (3.0304, -40.1222)
  line L12309 (2.4486, -39.2464) -> (2.6116, -39.3346)
  line L12310 (11.5439, -42.6665) -> (11.4027, -42.5464)
  line L12311 (6.8326, -39.0201) -> (7.1147, -39.0046)
  line L12312 (27.9001, -41.4537) -> (28.0845, -41.473)
  line L12313 (27.3733, -41.6087) -> (27.5376, -41.5228)
  line L12314 (6.5555, -39.0752) -> (6.8326, -39.0201)
  line L12315 (12.7601, -41.2171) -> (12.8773, -41.3607)
  line L12316 (1.4157, -39.4434) -> (1.5602, -39.3273)
  line L12317 (-10.0593, -38.8719) -> (-10.2411, -39.0881)
  line L12318 (-9.6774, -37.6963) -> (-9.6813, -37.8219)
  line L12319 (-10.3547, -36.1961) -> (-10.1565, -36.3974)
  line L12320 (-12.5853, -39.4783) -> (-12.8274, -39.3326)
  line L12321 (-13.3988, -38.7144) -> (-13.5251, -38.4617)
  line L12322 (-12.0521, -39.6609) -> (-12.3252, -39.5885)
  line L12323 (2.8567, -40.6698) -> (2.7355, -40.8102)
  line L12324 (-9.8545, -36.8733) -> (-9.7568, -37.1383)
  line L12325 (3.03, -40.1487) -> (3.0068, -40.3327)
  line L12326 (-13.6145, -38.1937) -> (-13.6653, -37.9158)
  line L12327 (-11.2105, -39.6411) -> (-11.4891, -39.6874)
  line L12328 (-13.5795, -37.0783) -> (-13.4734, -36.8164)
  line L12329 (-13.3315, -36.5722) -> (-13.1566, -36.3503)
  line L12330 (1.9024, -39.189) -> (2.087, -39.1722)
  line L12331 (-13.6764, -37.6335) -> (-13.6476, -37.3525)
  line L12332 (-13.1566, -36.3503) -> (-12.9522, -36.1553)
  line L12333 (2.2454, -41.0578) -> (2.0605, -41.072)
  line L12334 (12.5951, -42.6886) -> (12.4296, -42.7722)
  line L12335 (2.087, -39.1722) -> (2.2714, -39.1916)
  line L12336 (-9.9887, -36.6247) -> (-9.8545, -36.8733)
  line L12337 (1.1305, -40.1089) -> (1.1512, -39.9247)
  line L12338 (-10.2411, -39.0881) -> (-10.4515, -39.2766)
  line L12339 (-13.2382, -38.9468) -> (-13.3988, -38.7144)
  line L12340 (-12.3252, -39.5885) -> (-12.5853, -39.4783)
  line L12341 (-10.5793, -36.0247) -> (-10.3547, -36.1961)
  line L12342 (11.7302, -41.0056) -> (11.908, -40.9533)